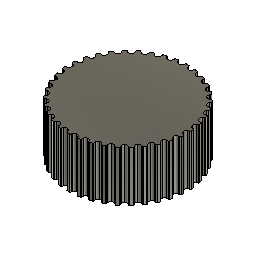
gear_38z (Autodesk Fusion 360 design; units mm, degrees)
Autodesk Fusion 360 part; units mm, degrees
sketch "Sketch1" plane through (0, 0, 0) normal (0, 0, 1) x (1, 0, 0) in component "gt2 pulley"
  circle A0 centre (0, 0) radius 12.0958 construction
  circle A1 centre (0, 0) radius 11.0918 construction
  line L0 (0, 0) -> (0, 12.0958) construction
  line L1 (0, 0) -> (0.9989, 12.0545) construction
  line L2 (0, 0) -> (1.4088, 12.0135) construction
  circle A2 centre (0, 0) radius 11.8418 construction
  arc A3 (0.3812, 11.6988) -> (0.4412, 11.4147) centre (1.3792, 11.7612) ccw
  circle A4 centre (0, 0) radius 11.6918 construction
  arc A5 (0.2344, 11.8395) -> (0, 11.8418) centre (0, 0) ccw
  arc A6 (0.3812, 11.6988) -> (0.2344, 11.8395) centre (0.2315, 11.6895) ccw
  arc A7 (0.4412, 11.4147) -> (0.916, 11.0539) centre (0.9618, 11.607) ccw
  arc A8 (0, 11.8418) -> (-0.2344, 11.8395) centre (0, 0) ccw
  arc A9 (-0.2344, 11.8395) -> (-0.3812, 11.6988) centre (-0.2315, 11.6895) ccw
  arc A10 (-0.4412, 11.4147) -> (-0.3812, 11.6988) centre (-1.3792, 11.7612) ccw
  arc A11 (-0.9157, 11.0539) -> (-0.4412, 11.4147) centre (-0.9618, 11.607) ccw
  arc A12 (0.916, 11.0539) -> (-0.916, 11.0539) centre (0, 0) ccw
  point P0 (1.3792, 11.7612)
  point P1 (0, 11.8418)
  dimension "d18" = 24.1916
  dimension "d19" = 4.737
  dimension "d22" = 1.004
  dimension "d24" = 0.75
  dimension "d26" = 1
  dimension "d27" = 0.15
  dimension "d28" = 0.15
  dimension "d47" = 0.555
  dimension "d52" = 3.812
  constraint coincident A0.centre A1.centre
  constraint coincident A0 L0.end
  constraint vertical L0
  constraint coincident A0 L1.end
  constraint coincident A0 L2.end
  constraint concentric A1 A2
  constraint coincident A1 A7.end
  constraint coincident L1 A7.end
  constraint coincident A2 P0
  constraint coincident L2 P0
  constraint coincident P0 A3.centre
  constraint coincident A2 P1
  constraint coincident L0 P1
  constraint concentric A2 A4
  constraint coincident P1 A5.end
  constraint coincident A4 A6.centre
  constraint coincident A3.start A6.start
  constraint tangent A3 A6
  constraint tangent A3 A7
  constraint symmetric L0 A7.end A12.end
  constraint symmetric L0 A3.start A9.end
  constraint symmetric L0 A3.end A10.start
  constraint symmetric L0 A3 A10
  constraint symmetric L0 A5.start A8.end
  constraint symmetric L0 P1 A5.end
  constraint symmetric L0 A5 A8
  constraint symmetric L0 A6 A9
  constraint symmetric L0 A7 A11
  constraint coincident A1 A11.start
  constraint tangent A1 A7
  constraint coincident L1 A7.centre
  measures "d18" diameter of A0
  measures "d19" angle of L0 L1
  measures "d22" distance of A0 A1
  measures "d24" distance of A1 A2
  measures "d26" radius of A3
  measures "d27" distance of A2 A4
  measures "d28" radius of A6
  measures "d47" radius of A7
extrude "Extrude1" add sketch "Sketch1" along normal blind 10 makes body 1
pattern_circular "C-Pattern1" count 38 over 360 about axis through (0, 0, 1.75) along (0, 0, 1) of bodies 1 makes body 2 at (-2.5247, 10.8006, 6.6667) makes body 3 at (-4.268, 10.2378, 6.6667) makes body 4 at (-5.1892, 9.8031, 6.6667) makes body 5 at (-6.2362, 9.1727, 3.3333) makes body 6 at (-8.0911, 7.587, 6.6667) makes body 7 at (-9.6562, 5.4576, 6.6667) makes body 8 at (-9.8502, 5.099, 3.3333) makes body 9 at (-10.5552, 3.4082, 3.3333) makes body 10 at (-11.0899, 0.204, 6.6667) makes body 11 at (-10.9722, -1.6241, 6.6667) makes body 12 at (-10.9051, -2.0263, 3.3333) makes body 13 at (-9.8504, -5.0988, 6.6667) makes body 14 at (-9.2296, -6.1516, 6.6667) makes body 15 at (-7.6611, -8.021, 6.6667) makes body 16 at (-6.8929, -8.69, 6.6667) makes body 17 at (-4.6416, -10.0739, 6.6667) makes body 18 at (-4.2682, -10.2377, 3.3333) makes body 19 at (-1.1191, -11.0352, 6.6667) makes body 20 at (-0.102, -11.0913, 6.6667) makes body 21 at (2.5247, -10.8006, 6.6667) makes body 22 at (4.268, -10.2378, 6.6667) makes body 23 at (4.6413, -10.074, 6.6667) makes body 24 at (7.3609, -8.2973, 6.6667) makes body 25 at (8.6262, -6.9725, 6.6667) makes body 26 at (8.8766, -6.6508, 3.3333) makes body 27 at (9.8502, -5.099, 3.3333) makes body 28 at (10.5552, -3.4082, 3.3333) makes body 29 at (10.9722, -1.6244, 3.3333) makes body 30 at (11.0899, 0.2037, 3.3333) makes body 31 at (10.9051, 2.0263, 6.6667) makes body 32 at (10.4229, 3.7936, 3.3333) makes body 33 at (9.3411, 5.981, 6.6667) makes body 34 at (7.6611, 8.021, 6.6667) makes body 35 at (6.2364, 9.1725, 6.6667) makes body 36 at (4.6416, 10.0739, 6.6667) makes body 37 at (4.2682, 10.2377, 3.3333) makes body 38 at (1.1191, 11.0352, 6.6667)
sketch "Sketch2" plane through (0, 0, 10) normal (0, 0, 1) x (-1, 0, 0)
  arc A0 (-10.8666, -4.3503) -> (-10.9364, -4.5412) centre (-10.7979, -4.4837) ccw
  arc A1 (-10.9364, -4.5412) -> (-10.7481, -4.9705) centre (0, 0) ccw
  arc A2 (-10.7481, -4.9705) -> (-10.5604, -5.0484) centre (-10.6119, -4.9076) ccw
  arc A3 (-10.2761, -4.9892) -> (-10.5604, -5.0484) centre (-10.2166, -5.9875) ccw
  arc A4 (-9.755, -5.2789) -> (-10.2761, -4.9892) centre (-10.243, -5.5433) ccw
  arc A5 (-10.4908, -3.6015) -> (-9.755, -5.2789) centre (0, 0) ccw
  arc A6 (-10.6305, -4.1812) -> (-10.4908, -3.6015) centre (-11.0157, -3.7817) ccw
  arc A7 (-10.8666, -4.3503) -> (-10.6305, -4.1812) centre (-11.3246, -3.4614) ccw
  circle A8 centre (0, 0) radius 11.0918
  constraint concentric A1 A8
extrude "Extrude2" add sketch "Sketch2" against normal blind 10 contours A5 A8 bodies 1 2 3 4 5 6 7 8 9 10 11 12 13 14 15 16 17 18 19 20 21 22 23 24 25 26 27 28 29 30 31 32 33 34 35 36 37 38
extrude "Extrude4" [suppressed] in component "gt2 pulley"
pattern_circular "C-Pattern7" [suppressed] in component "gt2 pulley"
extrude "Extrude3" [suppressed] in component "gt2 pulley"
pattern_circular "C-Pattern6" [suppressed] in component "gt2 pulley"
extrude "Extrude2'" [suppressed] in component "gt2 pulley"
pattern_circular "C-Pattern5" [suppressed] in component "gt2 pulley"
extrude "Extrude1'" [suppressed] in component "gt2 pulley"
pattern_circular "C-Pattern4" [suppressed] in component "gt2 pulley"
pattern_circular "C-Pattern3" [suppressed] in component "gt2 pulley"
pattern_circular "C-Pattern2" [suppressed] in component "gt2 pulley"
pattern_circular "C-Pattern1'" [suppressed] in component "gt2 pulley"
copy_body "Body->Comp1" [suppressed] in component "Component"
copy_body "Body->Comp2" [suppressed] in component "Component'"
copy_body "Body->Comp3" [suppressed] in component "Component''"
copy_body "Body->Comp4" [suppressed] in component "Component'''"
copy_body "Body->Comp5" [suppressed] in component "Component''''"
copy_body "Body->Comp6" [suppressed] in component "Component'''''"
copy_body "Body->Comp7" [suppressed] in component "Component''''''"
copy_body "Body->Comp8" [suppressed] in component "Component'''''''"
copy_body "Body->Comp9" [suppressed] in component "Component''''''''"
copy_body "Body->Comp10" [suppressed] in component "Component'''''''''"
copy_body "Body->Comp11" [suppressed] in component "Component''''''''''"
copy_body "Body->Comp12" [suppressed] in component "Component'''''''''''"
copy_body "Body->Comp13" [suppressed] in component "Component''''''''''''"
copy_body "Body->Comp14" [suppressed] in component "Component'''''''''''''"
copy_body "Body->Comp15" [suppressed] in component "Component''''''''''''''"
copy_body "Body->Comp16" [suppressed] in component "Component'''''''''''''''"
copy_body "Body->Comp17" [suppressed] in component "Component''''''''''''''''"
copy_body "Body->Comp18" [suppressed] in component "Component'''''''''''''''''"
copy_body "Body->Comp19" [suppressed] in component "Component''''''''''''''''''"
copy_body "Body->Comp20" [suppressed] in component "Component'''''''''''''''''''"
component "gt2 pulley" placed x (1, 0, 0) y (0, 1, 0) z (0, 0, 1) at (0, 0, 0)
equation "NumTeeth = 38" comment "min 20"
equation "ToothPitch = 2 mm"
equation "PullyDia = NumTeeth * ToothPitch / PI"
equation "ToothAng = ( ( 360 / NumTeeth ) * 1 deg )"
equation "TransOffsetAngle = ToothAng * 0.2"
equation "Sholulder_Radius = 0.15 mm"
equation "Root_Radius = 0.555 mm"
equation "TransRadius = 1 mm"
equation "ToolHeight = 0.75 mm"
equation "PLD = 0.254 mm"
equation "d18 = PullyDia"
equation "d19 = ToothAng / 2"
equation "d22 = PLD + ToolHeight"
equation "d24 = ToolHeight"
equation "d26 = TransRadius"
equation "d27 = Sholulder_Radius"
equation "d31 = NumTeeth"
equation "d33 = NumTeeth"
equation "d35 = NumTeeth"
equation "d37 = NumTeeth"
equation "d41 = NumTeeth"
equation "d45 = NumTeeth"
equation "d47 = Root_Radius"
equation "d50 = NumTeeth"
